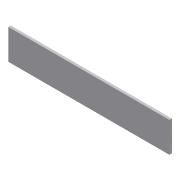
# Autodesk Inventor part: FE-00002-07
Saved by Autodesk Inventor 2012 (Build 160160000, 160)
## iProperties
Created: 2008-05-14
Part Number: FE-00002-07
Document SubType Name: Modeling
Designer: narosenberg
Density: 1 g/cm^3
Mass: 196.645 g
Surface Area: 680.644 cm^2
Volume: 196.645 cm^3
Material: Default
Author: narosenberg
Autodesk Inventor part; units mm, degrees
ref_plane "YZ Plane" through (0, 0, 0) normal (1, 0, 0) x (0, 1, 0)
ref_plane "XZ Plane" through (0, 0, 0) normal (0, 1, 0) x (-1, 0, 0)
sketch "Sketch1" plane through (0, 0, 0) normal (0, 0, 1) x (1, 0, 0)
  line L0 (-35.3081, 19.4313) -> (371.0919, 19.4313)
  line L1 (371.0919, 19.4313) -> (371.0919, -56.7687)
  line L2 (371.0919, -56.7687) -> (-35.3081, -56.7687)
  line L3 (-35.3081, -56.7687) -> (-35.3081, 19.4313)
  dimension "d0" = 406.4
  dimension "d1" = 76.2
  constraints: 8 end point, 2 parallel, 1 horizontal, 1 perpendicular
  measures "d0" distance of L0.start L0.end
  measures "d1" distance of L2.end L0.start
extrude "Extrusion1" add sketch "Sketch1" along normal blind 6.35
ref_plane "Work Plane2" through (-35.3081, -18.6687, 0) normal (0, 1, 0) x (1, 0, 0)
equation "\"d5\" = -0.5 * d1"
body "Solid1"
